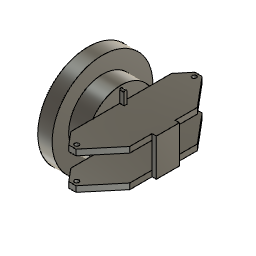
INDUSTRIAL ROBOT v3 (Autodesk Fusion 360 archive; units mm, degrees)
design "ITEM 3"
Autodesk Fusion 360 part; units mm, degrees
sketch "Sketch1" plane through (0, 0, 0) normal (1, 0, 0) x (0, 1, 0)
  circle A0 centre (0, 0) radius 35
  dimension "d1" = 70
  constraint coincident A0.centre origin
  measures "d1" diameter of A0
extrude "Extrude1" add sketch "Sketch1" along normal blind 10 in component "Component"
sketch "Sketch2" plane through (10, 0, 0) normal (1, 0, 0) x (0, 1, 0)
  circle A0 centre (0, 0) radius 35
  circle A1 centre (0, 0) radius 23.5
  dimension "d4" = 47
  constraint coincident A0.centre A1.centre
  measures "d4" diameter of A1
extrude "Extrude2" add sketch "Sketch2" along normal blind 13 contours A1 in component "Component"
ref_plane "WorkPlane1" through (0, 0, 13) normal (0, 0, 1) x (1, 0, 0)
sketch "Sketch3" plane through (0, 0, 13) normal (0, 0, 1) x (1, 0, 0)
  line L0 (23, 0) -> (23, -35)
  line L1 (23, -35) -> (23, -45)
  line L2 (23, -35) -> (30.3921, -43.8095)
  line L3 (23, -35) -> (34.5, -35) construction
  line L4 (23, 0) -> (60, 0)
  line L5 (23, -23.4992) -> (67, -23.4992)
  line L6 (30.3921, -43.8095) -> (35.3921, -43.8095)
  line L7 (35.3921, -43.8095) -> (52.4344, -23.4992)
  line L8 (35.3921, -43.8095) -> (45, -43.8095)
  line L9 (52.4344, -23.4992) -> (52.4344, 0)
  line L10 (23, 0) -> (23, 35)
  line L11 (23, 35) -> (30.3921, 43.8095)
  line L12 (30.3921, 43.8095) -> (35.3921, 43.8095)
  line L13 (52.4344, 23.4992) -> (52.4344, 0)
  line L14 (35.3921, 43.8095) -> (52.4344, 23.4992)
  dimension "d8" = 35
  dimension "d9" = 10
  dimension "d10" = 50
  dimension "d11" = 11.5
  dimension "d13" = 37
  dimension "d14" = 44
  dimension "d15" = 5
  dimension "d16" = 50
  constraint vertical L0
  constraint parallel L0 L1
  constraint horizontal L3
  constraint perpendicular L0 L4
  constraint coincident L0 L5.start
  constraint perpendicular L0 L5
  constraint horizontal L6
  constraint coincident L5 L7.end
  constraint parallel L5 L8
  constraint coincident L4 L9.end
  constraint perpendicular L4 L9
  constraint symmetric L0.start L4 L10.start
  constraint symmetric L0.end L4 L10.end
  constraint symmetric L2.end L4 L11.end
  constraint symmetric L4 L6.end L12.end
  constraint symmetric L4 L7.end L13.start
  constraint symmetric L4 L9.end L13.end
  measures "d8" distance of L0.start L0.end
  measures "d9" distance of L0.end L1.end
  measures "d10" angle of L2 L3
  measures "d11" distance of L0.end L2.end
  measures "d13" distance of L0.start L4.end
  measures "d14" distance of L5.start L5.end
  measures "d15" distance of L2.end L6.end
  measures "d16" angle of L7 L8
extrude "Extrude3" add sketch "Sketch3" against normal blind 4 in component "Component"
sketch "Sketch4" plane through (0, 0, 13) normal (0, 0, 1) x (-1, 0, 0)
  line L0 (-23, -35) -> (-23, -19.5768)
  line L1 (-23, -19.5768) -> (-23, 19.5768)
  line L2 (-23, 19.5768) -> (-23, 35)
  line L3 (-23, 35) -> (-30.3921, 43.8095)
  line L4 (-30.3921, 43.8095) -> (-35.3921, 43.8095)
  line L5 (-35.3921, 43.8095) -> (-52.4344, 23.4992)
  line L6 (-52.4344, 23.4992) -> (-52.4344, -23.4992)
  line L7 (-52.4344, -23.4992) -> (-35.3921, -43.8095)
  line L8 (-35.3921, -43.8095) -> (-30.3921, -43.8095)
  line L9 (-30.3921, -43.8095) -> (-23, -35)
  line L10 (-32.8921, 43.8095) -> (-32.8921, 40.8095)
  circle A0 centre (-32.8921, 40.8095) radius 1.5
  dimension "d19" = 3
  dimension "d20" = 3
  constraint midpoint L4 L10.start
  constraint perpendicular L4 L10
  constraint coincident L10.end A0.centre
  measures "d19" distance of L10.start L10.end
  measures "d20" diameter of A0
extrude "Extrude4" cut sketch "Sketch4" against normal blind 7 contours A0 in component "Component"
mirror "Mirror1" about plane through (0, 0, 0) normal (0, 1, 0) of "Extrude4" in component "Component"
mirror "Mirror2" about plane through (0, 0, 0) normal (0, 0, 1) of "Extrude3", "Extrude4", "Mirror1" in component "Component"
sketch "Sketch5" plane through (23, 0, 0) normal (1, 0, 0) x (0, 1, 0)
  line L0 (-19.5768, 13) -> (19.5768, 13)
  arc A0 (19.5768, 13) -> (-19.5768, 13) centre (0, 0) ccw
  line L1 (0, 13) -> (0, 23.5)
  line L2 (0, 13) -> (-1, 13)
  line L3 (-1, 13) -> (-1, 22)
  line L4 (-1, 22) -> (1, 22)
  line L5 (1, 22) -> (1, 13)
  constraint midpoint L0 L1.start
  constraint midpoint A0 L1.end
  constraint coincident L0 L2.end
  constraint perpendicular L2 L3
  constraint perpendicular L1 L4
  constraint coincident L0 L5.end
  constraint perpendicular L0 L5
extrude "Extrude5" add sketch "Sketch5" along normal blind 3 contours L0 L1 L2 L3 L4 | L0 L1 L4 L5 in component "Component"
fillet "Fillet1" radius 1 2 edges at (24.5, 1, 22) (24.5, -1, 22) in component "Component"
mirror "Mirror3" about plane through (0, 0, 0) normal (0, 0, 1) of "Extrude5", "Fillet1" in component "Component"
sketch "Sketch6" plane through (52.4344, 0, 0) normal (1, 0, 0) x (0, 1, 0)
  line L0 (23.4992, 13) -> (-23.4992, 13)
  line L1 (-23.4992, 13) -> (-23.4992, 9)
  line L2 (-23.4992, 9) -> (23.4992, 9)
  line L3 (23.4992, 9) -> (23.4992, 13)
  line L4 (8, -13) -> (-8, -13)
  line L5 (-8, -13) -> (-8, 13)
  line L6 (-8, 13) -> (8, 13)
  line L7 (8, 13) -> (8, -13)
  line L8 (8, -13) -> (-8, 13) construction
  line L9 (-8, -13) -> (8, 13) construction
  constraint horizontal L4
  constraint perpendicular L4 L5
  constraint parallel L4 L6
  constraint parallel L5 L7
  constraint coincident L8 origin
  constraint coincident L9 origin
extrude "Extrude6" add sketch "Sketch6" along normal blind 3 contours L0 L2 L5 L6 L7 | L2 L4 L5 L7 in component "Component"
sketch "Sketch7" plane through (0, 0, 0) normal (-1, 0, 0) x (0, -1, 0)
  circle A0 centre (0, 0) radius 35
  circle A1 centre (0, 0) radius 10
  dimension "d35" = 20
  constraint coincident A0.centre A1.centre
  measures "d35" diameter of A1
extrude "Extrude7" cut sketch "Sketch7" against normal blind 10 contours A1 in component "Component"
component "Component" placed x (1, 0, 0) y (0, 1, 0) z (0, 0, 1) at (0, 0, 0)

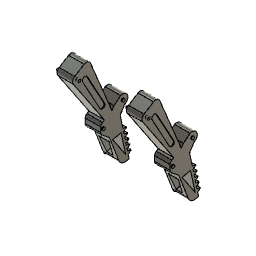
design "JAW FINAL"
Autodesk Fusion 360 part; units mm, degrees
sketch "Sketch1" plane through (0, 0, 0) normal (1, 0, 0) x (0, 1, 0)
  line L0 (308.6071, 26.1218) -> (329.0653, 38.6702)
  line L1 (329.0653, 38.6702) -> (356.1703, -26.9523)
  line L2 (364.0358, -80.7741) -> (365.4972, -87.6198)
  line L3 (365.4972, -87.6198) -> (376.2548, -85.3234)
  line L4 (376.2548, -85.3234) -> (365.8164, -36.4251)
  line L5 (365.8164, -36.4251) -> (371.2115, -28.0053)
  line L6 (308.6071, 26.1218) -> (347.5605, -32.0386)
  line L7 (356.1703, -26.9523) -> (347.5605, -32.0386)
  line L8 (347.5605, -32.0386) -> (343.2556, -34.5818)
  line L9 (343.2556, -34.5818) -> (343.2556, -44.5818)
  line L10 (343.2556, -44.5818) -> (353.387, -52.7276)
  line L11 (343.2556, -44.5818) -> (352.5031, -44.5818) construction
  line L12 (353.387, -52.7276) -> (364.0358, -80.7741)
  line L13 (356.1703, -26.9523) -> (358.6771, -23.3241)
  line L14 (358.6771, -23.3241) -> (366.4246, -17.0014)
  arc A0 (371.2115, -28.0053) -> (363.9076, -19.0555) centre (368.8181, -22.5033) ccw
  dimension "d6" = 70
  dimension "d7" = 24
  dimension "d8" = 71
  dimension "d10" = 10
  dimension "d11" = 5
  dimension "d12" = 10
  dimension "d13" = 13
  dimension "d14" = 38.8
  dimension "d15" = 30
  dimension "d16" = 7
  dimension "d17" = 11
  dimension "d18" = 50
  dimension "d19" = 10
  dimension "d20" = 4.41
  dimension "d21" = 10
  dimension "d22" = 12
  constraint perpendicular L2 L3
  constraint perpendicular L3 L4
  constraint parallel L7 L8
  constraint vertical L9
  constraint horizontal L11
  constraint coincident L14.end A0
  constraint coincident L14 A0.end
  measures "d6" distance of L0.start L6.end
  measures "d7" distance of L0.start L0.end
  measures "d8" distance of L0.end L1.end
  measures "d10" distance of L1.end L6.end
  measures "d11" distance of L6.end L8.end
  measures "d12" distance of L8.end L9.end
  measures "d13" distance of L9.end L10.end
  measures "d14" angle of L10 L11
  measures "d15" distance of L2.start L10.end
  measures "d16" distance of L2.start L2.end
  measures "d17" distance of L2.end L3.end
  measures "d18" distance of L3.end L4.end
  measures "d19" distance of L4.end L5.end
  measures "d20" distance of L1.end L13.end
  measures "d21" distance of L13.end L14.end
  measures "d22" distance of L5.end L14.end
extrude "Extrude1" add sketch "Sketch1" along normal mid plane 18 contours L0 L1 L6 L7 | L2 L3 L4 L5 L7 L8 L9 L10 L12 L13 L14 A0 in component "Component"
sketch "Sketch2" plane through (-9, 0, 0) normal (-1, 0, 0) x (0, -1, 0)
  line L0 (-347.5605, -32.0386) -> (-308.6071, 26.1218)
  line L1 (-308.6071, 26.1218) -> (-329.0653, 38.6702)
  line L2 (-329.0653, 38.6702) -> (-356.1703, -26.9523)
  line L3 (-356.1703, -26.9523) -> (-358.6771, -23.3241)
  line L4 (-358.6771, -23.3241) -> (-366.4246, -17.0014)
  arc A0 (-366.4246, -17.0014) -> (-371.2115, -28.0053) centre (-368.8181, -22.5033) ccw
  line L5 (-371.2115, -28.0053) -> (-365.8164, -36.4251)
  line L6 (-365.8164, -36.4251) -> (-376.2548, -85.3234)
  line L7 (-376.2548, -85.3234) -> (-365.4972, -87.6198)
  line L8 (-365.4972, -87.6198) -> (-364.0358, -80.7741)
  line L9 (-364.0358, -80.7741) -> (-353.387, -52.7276)
  line L10 (-353.387, -52.7276) -> (-343.2556, -44.5818)
  line L11 (-343.2556, -44.5818) -> (-343.2556, -34.5818)
  line L12 (-343.2556, -34.5818) -> (-347.5605, -32.0386)
sketch "Sketch3" plane through (9, 0, 0) normal (1, 0, 0) x (0, 1, 0)
  line L0 (308.6071, 26.1218) -> (347.5605, -32.0386)
  line L1 (347.5605, -32.0386) -> (343.2556, -34.5818)
  line L2 (343.2556, -34.5818) -> (343.2556, -44.5818)
  line L3 (343.2556, -44.5818) -> (353.387, -52.7276)
  line L4 (353.387, -52.7276) -> (364.0358, -80.7741)
  line L5 (364.0358, -80.7741) -> (365.4972, -87.6198)
  line L6 (365.4972, -87.6198) -> (376.2548, -85.3234)
  line L7 (376.2548, -85.3234) -> (365.8164, -36.4251)
  line L8 (365.8164, -36.4251) -> (371.2115, -28.0053)
  arc A0 (371.2115, -28.0053) -> (366.4246, -17.0014) centre (368.8181, -22.5033) ccw
  line L9 (366.4246, -17.0014) -> (358.6771, -23.3241)
  line L10 (358.6771, -23.3241) -> (356.1703, -26.9523)
  line L11 (356.1703, -26.9523) -> (329.0653, 38.6702)
  line L12 (329.0653, 38.6702) -> (308.6071, 26.1218)
  line L13 (364.0358, -80.7741) -> (372.1529, -79.0413)
  line L14 (372.1529, -79.0413) -> (366.9337, -54.5922)
  line L15 (372.1529, -79.0413) -> (366.9337, -54.5922)
  line L16 (366.9337, -54.5922) -> (357.1541, -56.6798)
  line L17 (357.1541, -56.6798) -> (372.1529, -79.0413)
  dimension "d25" = 90
  dimension "d26" = 25
  dimension "d28" = 2.7
  dimension "d29" = 10
  constraint coincident L4.end L5.start
  constraint perpendicular L5 L13
  constraint perpendicular L14 L16
  measures "d25" angle of L13 L14
  measures "d26" distance of L13.end L14.end
  measures "d28" distance of L7 L15
  measures "d29" distance of L14.end L16.end
extrude "Extrude2" cut sketch "Sketch3" against normal blind 68 contours L14 L15 L16 L17 in component "Component"
sketch "Sketch4" plane through (9, 0, 0) normal (1, 0, 0) x (0, 1, 0)
  line L0 (366.9337, -54.5922) -> (372.1529, -79.0413)
  line L1 (372.1529, -79.0413) -> (357.1541, -56.6798)
  line L2 (357.1541, -56.6798) -> (366.9337, -54.5922)
  line L3 (308.6071, 26.1218) -> (347.5605, -32.0386)
  line L4 (347.5605, -32.0386) -> (343.2556, -34.5818)
  line L5 (343.2556, -34.5818) -> (343.2556, -44.5818)
  line L6 (343.2556, -44.5818) -> (353.387, -52.7276)
  line L7 (353.387, -52.7276) -> (364.0358, -80.7741)
  line L8 (364.0358, -80.7741) -> (365.4972, -87.6198)
  line L9 (365.4972, -87.6198) -> (376.2548, -85.3234)
  line L10 (376.2548, -85.3234) -> (365.8164, -36.4251)
  line L11 (365.8164, -36.4251) -> (371.2115, -28.0053)
  arc A0 (371.2115, -28.0053) -> (366.4246, -17.0014) centre (368.8181, -22.5033) ccw
  line L12 (366.4246, -17.0014) -> (358.6771, -23.3241)
  line L13 (358.6771, -23.3241) -> (356.1703, -26.9523)
  line L14 (356.1703, -26.9523) -> (329.0653, 38.6702)
  line L15 (329.0653, 38.6702) -> (308.6071, 26.1218)
  line L16 (376.2548, -85.3234) -> (375.2109, -80.4336)
  line L17 (375.2109, -80.4336) -> (374.3759, -76.5217)
  line L18 (374.7934, -78.4776) -> (378.7053, -77.6426)
  line L19 (378.7053, -77.6426) -> (374.3759, -76.5217)
  line L20 (375.2109, -80.4336) -> (378.7053, -77.6426)
  line L21 (373.854, -74.0768) -> (377.3483, -71.2858)
  line L22 (373.4364, -72.1208) -> (377.3483, -71.2858)
  line L23 (377.3483, -71.2858) -> (373.0189, -70.1649)
  line L24 (373.854, -74.0768) -> (373.0189, -70.1649)
  line L25 (372.497, -67.72) -> (375.9913, -64.929)
  line L26 (372.0794, -65.7641) -> (375.9913, -64.929)
  line L27 (375.9913, -64.929) -> (371.6619, -63.8081)
  line L28 (372.497, -67.72) -> (371.6619, -63.8081)
  line L29 (371.14, -61.3632) -> (374.6343, -58.5722)
  line L30 (370.7225, -59.4073) -> (374.6343, -58.5722)
  line L31 (374.6343, -58.5722) -> (370.3049, -57.4514)
  line L32 (371.14, -61.3632) -> (370.3049, -57.4514)
  line L33 (369.783, -55.0065) -> (373.2773, -52.2155)
  line L34 (369.3655, -53.0505) -> (373.2773, -52.2155)
  line L35 (373.2773, -52.2155) -> (368.9479, -51.0946)
  line L36 (369.783, -55.0065) -> (368.9479, -51.0946)
  dimension "d32" = 5
  dimension "d33" = 4
  dimension "d34" = 4
  dimension "d37" = 26
  dimension "d38" = 0
  constraint coincident L9.end L10.start
  constraint perpendicular L9 L16
  constraint perpendicular L9 L17
  constraint midpoint L17 L18.start
  constraint perpendicular L17 L18
  measures "d32" distance of L9.end L16.end
  measures "d33" distance of L16.end L17.end
  measures "d34" distance of L18.start L18.end
extrude "Extrude3" add sketch "Sketch4" against normal up to surface (18 mm away) contours L10 L34 L35 L36 | L10 L17 L18 L20 | L10 L33 L34 L36 | L10 L17 L18 L19 | L10 L30 L31 L32 | L10 L21 L22 L24 | L10 L29 L30 L32 | L10 L22 L23 L24 | L10 L26 L27 L28 | L10 L25 L26 L28 in component "Component"
fillet "Fillet1" radius 5 2 edges at (0, 308.6071, 26.1218) (0, 329.0653, 38.6702) in component "Component"
fillet "Fillet2" radius 7.5 1 edges at (0, 365.4972, -87.6198) in component "Component"
fillet "Fillet3" radius 4 2 edges at (0, 343.2556, -44.5818) (0, 343.2556, -34.5818) in component "Component"
sketch "Sketch5" plane through (9, 0, 0) normal (1, 0, 0) x (0, 1, 0)
  arc A0 (345.221, -33.4207) -> (343.2556, -36.8646) centre (347.2556, -36.8646) ccw
  line L0 (343.2556, -36.8646) -> (343.2556, -42.6653)
  arc A1 (343.2556, -42.6653) -> (344.7491, -45.7827) centre (347.2556, -42.6653) ccw
  line L1 (344.7491, -45.7827) -> (353.387, -52.7276)
  line L2 (353.387, -52.7276) -> (364.0358, -80.7741)
  arc A2 (364.0358, -80.7741) -> (372.8156, -86.0576) centre (371.2498, -78.7228) ccw
  line L3 (372.8156, -86.0576) -> (376.2548, -85.3234)
  line L4 (376.2548, -85.3234) -> (375.2109, -80.4336)
  line L5 (375.2109, -80.4336) -> (378.7053, -77.6426)
  line L6 (378.7053, -77.6426) -> (374.3759, -76.5217)
  line L7 (374.3759, -76.5217) -> (373.854, -74.0768)
  line L8 (373.854, -74.0768) -> (377.3483, -71.2858)
  line L9 (377.3483, -71.2858) -> (373.0189, -70.1649)
  line L10 (373.0189, -70.1649) -> (372.497, -67.72)
  line L11 (372.497, -67.72) -> (375.9913, -64.929)
  line L12 (375.9913, -64.929) -> (371.6619, -63.8081)
  line L13 (371.6619, -63.8081) -> (371.14, -61.3632)
  line L14 (371.14, -61.3632) -> (374.6343, -58.5722)
  line L15 (374.6343, -58.5722) -> (370.3049, -57.4514)
  line L16 (370.3049, -57.4514) -> (369.783, -55.0065)
  line L17 (369.783, -55.0065) -> (373.2773, -52.2155)
  line L18 (373.2773, -52.2155) -> (368.9479, -51.0946)
  line L19 (368.9479, -51.0946) -> (365.8164, -36.4251)
  line L20 (365.8164, -36.4251) -> (371.2115, -28.0053)
  arc A3 (371.2115, -28.0053) -> (366.4246, -17.0014) centre (368.8181, -22.5033) ccw
  line L21 (366.4246, -17.0014) -> (358.6771, -23.3241)
  line L22 (358.6771, -23.3241) -> (356.1703, -26.9523)
  line L23 (356.1703, -26.9523) -> (331.3034, 33.2516)
  arc A4 (331.3034, 33.2516) -> (324.0678, 35.6049) centre (326.6821, 31.3428) ccw
  line L24 (324.0678, 35.6049) -> (313.043, 28.8426)
  arc A5 (313.043, 28.8426) -> (311.5029, 21.7981) centre (315.6572, 24.5805) ccw
  line L25 (311.5029, 21.7981) -> (347.5605, -32.0386)
  line L26 (347.5605, -32.0386) -> (345.221, -33.4207)
  line L27 (366.9337, -54.5922) -> (372.1529, -79.0413)
  line L28 (372.1529, -79.0413) -> (357.1541, -56.6798)
  line L29 (357.1541, -56.6798) -> (366.9337, -54.5922)
  circle A6 centre (314.3303, 24.5805) radius 1.5
  dimension "d49" = 3
  measures "d49" diameter of A6
extrude "Extrude4" cut sketch "Sketch5" against normal blind 29 contours A6 in component "Component"
sketch "Sketch6" plane through (0, 291.3636, 110.6267) normal (0, -0.934881, -0.354961) x (1, 0, 0)
  line L0 (-9, -204.7328) -> (9, -204.7328)
  line L1 (9, -204.7328) -> (9, -174.7328)
  line L2 (9, -174.7328) -> (-9, -174.7328)
  line L3 (-9, -174.7328) -> (-9, -204.7328)
  line L4 (-6, -182.1738) -> (6, -182.1738)
  line L5 (-7, -201.7782) -> (3.528, -201.7782)
  line L6 (3.528, -201.7782) -> (6, -182.1738)
  line L7 (-6, -182.1738) -> (-3.4614, -201.7782)
  dimension "d52" = 3
  dimension "d53" = 3
  dimension "d54" = 7.441
  constraint horizontal L4
  constraint horizontal L5
  constraint coincident L5 L7.end
  measures "d52" distance of L1 L4.end
  measures "d53" distance of L3 L4.start
  measures "d54" distance of L2 L4
extrude "Extrude5" cut sketch "Sketch6" against normal blind 8 contours L4 L5 L6 L7 in component "Component"
sketch "Sketch7" plane through (9, 0, 0) normal (1, 0, 0) x (0, 1, 0)
  circle A0 centre (314.3303, 24.5805) radius 1.5
  arc A1 (345.221, -33.4207) -> (343.2556, -36.8646) centre (347.2556, -36.8646) ccw
  line L0 (343.2556, -36.8646) -> (343.2556, -42.6653)
  arc A2 (343.2556, -42.6653) -> (344.7491, -45.7827) centre (347.2556, -42.6653) ccw
  line L1 (344.7491, -45.7827) -> (353.387, -52.7276)
  line L2 (353.387, -52.7276) -> (364.0358, -80.7741)
  arc A3 (364.0358, -80.7741) -> (372.8156, -86.0576) centre (371.2498, -78.7228) ccw
  line L3 (372.8156, -86.0576) -> (376.2548, -85.3234)
  line L4 (376.2548, -85.3234) -> (375.2109, -80.4336)
  line L5 (375.2109, -80.4336) -> (378.7053, -77.6426)
  line L6 (378.7053, -77.6426) -> (374.3759, -76.5217)
  line L7 (374.3759, -76.5217) -> (373.854, -74.0768)
  line L8 (373.854, -74.0768) -> (377.3483, -71.2858)
  line L9 (377.3483, -71.2858) -> (373.0189, -70.1649)
  line L10 (373.0189, -70.1649) -> (372.497, -67.72)
  line L11 (372.497, -67.72) -> (375.9913, -64.929)
  line L12 (375.9913, -64.929) -> (371.6619, -63.8081)
  line L13 (371.6619, -63.8081) -> (371.14, -61.3632)
  line L14 (371.14, -61.3632) -> (374.6343, -58.5722)
  line L15 (374.6343, -58.5722) -> (370.3049, -57.4514)
  line L16 (370.3049, -57.4514) -> (369.783, -55.0065)
  line L17 (369.783, -55.0065) -> (373.2773, -52.2155)
  line L18 (373.2773, -52.2155) -> (368.9479, -51.0946)
  line L19 (368.9479, -51.0946) -> (365.8164, -36.4251)
  line L20 (365.8164, -36.4251) -> (371.2115, -28.0053)
  arc A4 (371.2115, -28.0053) -> (366.4246, -17.0014) centre (368.8181, -22.5033) ccw
  line L21 (366.4246, -17.0014) -> (358.6771, -23.3241)
  line L22 (358.6771, -23.3241) -> (356.1703, -26.9523)
  line L23 (356.1703, -26.9523) -> (331.3034, 33.2516)
  arc A5 (331.3034, 33.2516) -> (324.0678, 35.6049) centre (326.6821, 31.3428) ccw
  line L24 (324.0678, 35.6049) -> (313.043, 28.8426)
  arc A6 (313.043, 28.8426) -> (311.5029, 21.7981) centre (315.6572, 24.5805) ccw
  line L25 (311.5029, 21.7981) -> (347.5605, -32.0386)
  line L26 (347.5605, -32.0386) -> (345.221, -33.4207)
  line L27 (366.9337, -54.5922) -> (372.1529, -79.0413)
  line L28 (372.1529, -79.0413) -> (357.1541, -56.6798)
  line L29 (357.1541, -56.6798) -> (366.9337, -54.5922)
  circle A7 centre (368.8181, -22.5033) radius 1.75
  circle A8 centre (345.9618, -39.765) radius 1.75
  dimension "d57" = 3.5
  dimension "d58" = 3.5
  constraint concentric A4 A7
  measures "d57" diameter of A7
  measures "d58" diameter of A8
extrude "Extrude6" add sketch "Sketch7" along normal blind 1 contours A7 | A8 in component "Component"
sketch "Sketch8" plane through (9, 0, 0) normal (1, 0, 0) x (0, 1, 0)
  circle A0 centre (368.8181, -22.5033) radius 1.75
  circle A1 centre (345.9618, -39.765) radius 1.75
  circle A2 centre (314.3303, 24.5805) radius 1.5
  arc A3 (345.221, -33.4207) -> (343.2556, -36.8646) centre (347.2556, -36.8646) ccw
  line L0 (343.2556, -36.8646) -> (343.2556, -42.6653)
  arc A4 (343.2556, -42.6653) -> (344.7491, -45.7827) centre (347.2556, -42.6653) ccw
  line L1 (344.7491, -45.7827) -> (353.387, -52.7276)
  line L2 (353.387, -52.7276) -> (364.0358, -80.7741)
  arc A5 (364.0358, -80.7741) -> (372.8156, -86.0576) centre (371.2498, -78.7228) ccw
  line L3 (372.8156, -86.0576) -> (376.2548, -85.3234)
  line L4 (376.2548, -85.3234) -> (375.2109, -80.4336)
  line L5 (375.2109, -80.4336) -> (378.7053, -77.6426)
  line L6 (378.7053, -77.6426) -> (374.3759, -76.5217)
  line L7 (374.3759, -76.5217) -> (373.854, -74.0768)
  line L8 (373.854, -74.0768) -> (377.3483, -71.2858)
  line L9 (377.3483, -71.2858) -> (373.0189, -70.1649)
  line L10 (373.0189, -70.1649) -> (372.497, -67.72)
  line L11 (372.497, -67.72) -> (375.9913, -64.929)
  line L12 (375.9913, -64.929) -> (371.6619, -63.8081)
  line L13 (371.6619, -63.8081) -> (371.14, -61.3632)
  line L14 (371.14, -61.3632) -> (374.6343, -58.5722)
  line L15 (374.6343, -58.5722) -> (370.3049, -57.4514)
  line L16 (370.3049, -57.4514) -> (369.783, -55.0065)
  line L17 (369.783, -55.0065) -> (373.2773, -52.2155)
  line L18 (373.2773, -52.2155) -> (368.9479, -51.0946)
  line L19 (368.9479, -51.0946) -> (365.8164, -36.4251)
  line L20 (365.8164, -36.4251) -> (371.2115, -28.0053)
  arc A6 (371.2115, -28.0053) -> (366.4246, -17.0014) centre (368.8181, -22.5033) ccw
  line L21 (366.4246, -17.0014) -> (358.6771, -23.3241)
  line L22 (358.6771, -23.3241) -> (356.1703, -26.9523)
  line L23 (356.1703, -26.9523) -> (331.3034, 33.2516)
  arc A7 (331.3034, 33.2516) -> (324.0678, 35.6049) centre (326.6821, 31.3428) ccw
  line L24 (324.0678, 35.6049) -> (313.043, 28.8426)
  arc A8 (313.043, 28.8426) -> (311.5029, 21.7981) centre (315.6572, 24.5805) ccw
  line L25 (311.5029, 21.7981) -> (347.5605, -32.0386)
  line L26 (347.5605, -32.0386) -> (345.221, -33.4207)
  line L27 (366.9337, -54.5922) -> (372.1529, -79.0413)
  line L28 (372.1529, -79.0413) -> (357.1541, -56.6798)
  line L29 (357.1541, -56.6798) -> (366.9337, -54.5922)
  line L30 (322.3738, 18.5661) -> (342.5242, -18.3398)
  arc A9 (342.5242, -18.3398) -> (347.7767, -15.4719) centre (345.1504, -16.9058) ccw
  line L31 (347.7767, -15.4719) -> (327.6262, 21.4339)
  arc A10 (327.6262, 21.4339) -> (322.3738, 18.5661) centre (325, 20) ccw
  line L32 (325, 20) -> (345.1504, -16.9058) construction
  constraint tangent L30 A9
  constraint tangent A9 L31
  constraint parallel L30 L31
  constraint tangent L31 A10
  constraint tangent L30 A10
extrude "Extrude7" cut sketch "Sketch8" against normal blind 1 contours L30 A9 L31 A10 in component "Component"
mirror "Mirror1" about plane through (0, 344.5115, -25.3555) normal (1, 0, 0) of "Extrude6", "Extrude7" in component "Component"
sketch "Sketch9" plane through (9, 0, 0) normal (1, 0, 0) x (0, 1, 0)
  line L0 (342.5242, -18.3398) -> (322.3738, 18.5661)
  arc A0 (327.6262, 21.4339) -> (322.3738, 18.5661) centre (325, 20) ccw
  line L1 (327.6262, 21.4339) -> (347.7767, -15.4719)
  arc A1 (342.5242, -18.3398) -> (347.7767, -15.4719) centre (345.1504, -16.9058) ccw
  circle A2 centre (368.8181, -22.5033) radius 1.75
  circle A3 centre (345.9618, -39.765) radius 1.75
  circle A4 centre (314.3303, 24.5805) radius 1.5
  arc A5 (345.221, -33.4207) -> (343.2556, -36.8646) centre (347.2556, -36.8646) ccw
  line L2 (343.2556, -36.8646) -> (343.2556, -42.6653)
  arc A6 (343.2556, -42.6653) -> (344.7491, -45.7827) centre (347.2556, -42.6653) ccw
  line L3 (344.7491, -45.7827) -> (353.387, -52.7276)
  line L4 (353.387, -52.7276) -> (364.0358, -80.7741)
  arc A7 (364.0358, -80.7741) -> (372.8156, -86.0576) centre (371.2498, -78.7228) ccw
  line L5 (372.8156, -86.0576) -> (376.2548, -85.3234)
  line L6 (376.2548, -85.3234) -> (375.2109, -80.4336)
  line L7 (375.2109, -80.4336) -> (378.7053, -77.6426)
  line L8 (378.7053, -77.6426) -> (374.3759, -76.5217)
  line L9 (374.3759, -76.5217) -> (373.854, -74.0768)
  line L10 (373.854, -74.0768) -> (377.3483, -71.2858)
  line L11 (377.3483, -71.2858) -> (373.0189, -70.1649)
  line L12 (373.0189, -70.1649) -> (372.497, -67.72)
  line L13 (372.497, -67.72) -> (375.9913, -64.929)
  line L14 (375.9913, -64.929) -> (371.6619, -63.8081)
  line L15 (371.6619, -63.8081) -> (371.14, -61.3632)
  line L16 (371.14, -61.3632) -> (374.6343, -58.5722)
  line L17 (374.6343, -58.5722) -> (370.3049, -57.4514)
  line L18 (370.3049, -57.4514) -> (369.783, -55.0065)
  line L19 (369.783, -55.0065) -> (373.2773, -52.2155)
  line L20 (373.2773, -52.2155) -> (368.9479, -51.0946)
  line L21 (368.9479, -51.0946) -> (365.8164, -36.4251)
  line L22 (365.8164, -36.4251) -> (371.2115, -28.0053)
  arc A8 (371.2115, -28.0053) -> (366.4246, -17.0014) centre (368.8181, -22.5033) ccw
  line L23 (366.4246, -17.0014) -> (358.6771, -23.3241)
  line L24 (358.6771, -23.3241) -> (356.1703, -26.9523)
  line L25 (356.1703, -26.9523) -> (331.3034, 33.2516)
  arc A9 (331.3034, 33.2516) -> (324.0678, 35.6049) centre (326.6821, 31.3428) ccw
  line L26 (324.0678, 35.6049) -> (313.043, 28.8426)
  arc A10 (313.043, 28.8426) -> (311.5029, 21.7981) centre (315.6572, 24.5805) ccw
  line L27 (311.5029, 21.7981) -> (347.5605, -32.0386)
  line L28 (347.5605, -32.0386) -> (345.221, -33.4207)
  line L29 (366.9337, -54.5922) -> (372.1529, -79.0413)
  line L30 (372.1529, -79.0413) -> (357.1541, -56.6798)
  line L31 (357.1541, -56.6798) -> (366.9337, -54.5922)
  circle A11 centre (314.3303, 24.5805) radius 1.5
  constraint concentric A4 A11
extrude "Extrude8" add sketch "Sketch9" against normal blind 21 contours A4 A11 in component "Component"
sketch "Sketch10" plane through (9, 0, 0) normal (1, 0, 0) x (0, 1, 0)
  line L0 (342.5242, -18.3398) -> (322.3738, 18.5661)
  arc A0 (327.6262, 21.4339) -> (322.3738, 18.5661) centre (325, 20) ccw
  line L1 (327.6262, 21.4339) -> (347.7767, -15.4719)
  arc A1 (342.5242, -18.3398) -> (347.7767, -15.4719) centre (345.1504, -16.9058) ccw
  circle A2 centre (368.8181, -22.5033) radius 1.75
  circle A3 centre (345.9618, -39.765) radius 1.75
  arc A4 (345.221, -33.4207) -> (343.2556, -36.8646) centre (347.2556, -36.8646) ccw
  line L2 (343.2556, -36.8646) -> (343.2556, -42.6653)
  arc A5 (343.2556, -42.6653) -> (344.7491, -45.7827) centre (347.2556, -42.6653) ccw
  line L3 (344.7491, -45.7827) -> (353.387, -52.7276)
  line L4 (353.387, -52.7276) -> (364.0358, -80.7741)
  arc A6 (364.0358, -80.7741) -> (372.8156, -86.0576) centre (371.2498, -78.7228) ccw
  line L5 (372.8156, -86.0576) -> (376.2548, -85.3234)
  line L6 (376.2548, -85.3234) -> (375.2109, -80.4336)
  line L7 (375.2109, -80.4336) -> (378.7053, -77.6426)
  line L8 (378.7053, -77.6426) -> (374.3759, -76.5217)
  line L9 (374.3759, -76.5217) -> (373.854, -74.0768)
  line L10 (373.854, -74.0768) -> (377.3483, -71.2858)
  line L11 (377.3483, -71.2858) -> (373.0189, -70.1649)
  line L12 (373.0189, -70.1649) -> (372.497, -67.72)
  line L13 (372.497, -67.72) -> (375.9913, -64.929)
  line L14 (375.9913, -64.929) -> (371.6619, -63.8081)
  line L15 (371.6619, -63.8081) -> (371.14, -61.3632)
  line L16 (371.14, -61.3632) -> (374.6343, -58.5722)
  line L17 (374.6343, -58.5722) -> (370.3049, -57.4514)
  line L18 (370.3049, -57.4514) -> (369.783, -55.0065)
  line L19 (369.783, -55.0065) -> (373.2773, -52.2155)
  line L20 (373.2773, -52.2155) -> (368.9479, -51.0946)
  line L21 (368.9479, -51.0946) -> (365.8164, -36.4251)
  line L22 (365.8164, -36.4251) -> (371.2115, -28.0053)
  arc A7 (371.2115, -28.0053) -> (366.4246, -17.0014) centre (368.8181, -22.5033) ccw
  line L23 (366.4246, -17.0014) -> (358.6771, -23.3241)
  line L24 (358.6771, -23.3241) -> (356.1703, -26.9523)
  line L25 (356.1703, -26.9523) -> (331.3034, 33.2516)
  arc A8 (331.3034, 33.2516) -> (324.0678, 35.6049) centre (326.6821, 31.3428) ccw
  line L26 (324.0678, 35.6049) -> (313.043, 28.8426)
  arc A9 (313.043, 28.8426) -> (311.5029, 21.7981) centre (315.6572, 24.5805) ccw
  line L27 (311.5029, 21.7981) -> (347.5605, -32.0386)
  line L28 (347.5605, -32.0386) -> (345.221, -33.4207)
  line L29 (366.9337, -54.5922) -> (372.1529, -79.0413)
  line L30 (372.1529, -79.0413) -> (357.1541, -56.6798)
  line L31 (357.1541, -56.6798) -> (366.9337, -54.5922)
  circle A10 centre (315.6572, 24.5805) radius 1.5
  dimension "d67" = 3
  constraint concentric A9 A10
  measures "d67" diameter of A10
extrude "Extrude9" add sketch "Sketch10" along normal blind 3 contours A10 in component "Component"
sketch "Sketch11" plane through (-12, 0, 0) normal (-1, 0, 0) x (0, -1, 0)
  circle A0 centre (-314.3303, 24.5805) radius 1.5
component "Component" placed x (1, 0, 0) y (0, 1, 0) z (0, 0, 1) at (0, 0, 0)
component "Component" placed x (1, 0, 0) y (0, 1, 0) z (0, 0, 1) at (52.854, 27.602, -25.252)

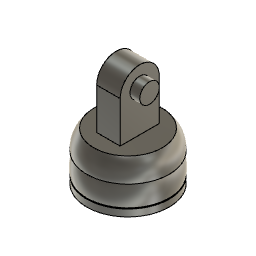
design "ITEM 2"
Autodesk Fusion 360 part; units mm, degrees
sketch "Sketch1" plane through (0, 0, 0) normal (0, 1, 0) x (1, 0, 0)
  line L0 (0, 0) -> (-35, 0)
  line L1 (0, 0) -> (0, 20)
  line L2 (0, 20) -> (-42, 20)
  arc A0 (-42, 20) -> (-35, 0) centre (-17.1273, 17.4804) ccw
  dimension "d1" = 35
  dimension "d2" = 20
  dimension "d3" = 42
  dimension "d4" = 25
  constraint coincident L0.start L1.start
  constraint horizontal L0
  constraint vertical L1
  constraint perpendicular L1 L2
  measures "d1" distance of L0.start L0.end
  measures "d2" distance of L0.start L1.end
  measures "d3" distance of L1.end L2.end
  measures "d4" radius of A0
revolve "Revolve1" add sketch "Sketch1" angle 360 about axis through (0, 0, 0) along (0, 0, -1) in component "Component"
sketch "Sketch2" plane through (0, 0, -20) normal (0, 0, -1) x (1, 0, 0)
  circle A0 centre (0, 0) radius 42
  circle A1 centre (0, 0) radius 39.5
  dimension "d6" = 79
  constraint coincident A0.centre A1.centre
  measures "d6" diameter of A1
extrude "Extrude1" add sketch "Sketch2" along normal blind 1 contours A1 in component "Component"
sketch "Sketch3" plane through (0, 0, 0) normal (1, 0, 0) x (0, 1, 0)
  line L0 (0, -21) -> (0, -41)
  line L1 (0, -41) -> (-42, -41)
  line L2 (0, -21) -> (-40, -21)
  arc A0 (-40, -21) -> (-42, -41) centre (-5.5677, -34.5432) ccw
  dimension "d9" = 20
  dimension "d10" = 42
  dimension "d11" = 40
  dimension "d12" = 37
  constraint vertical L0
  constraint perpendicular L0 L1
  constraint perpendicular L0 L2
  measures "d9" distance of L0.start L0.end
  measures "d10" distance of L0.end L1.end
  measures "d11" distance of L0.start L2.end
  measures "d12" radius of A0
revolve "Revolve2" add sketch "Sketch3" angle 360 about axis through (0, 0, -21) along (0, 0, -1) in component "Component"
sketch "Sketch4" plane through (0, 0, -41) normal (0, 0, -1) x (1, 0, 0)
  circle A0 centre (0, 0) radius 42
  circle A1 centre (0, 0) radius 41
  dimension "d14" = 82
  constraint coincident A0.centre A1.centre
  measures "d14" diameter of A1
extrude "Extrude2" add sketch "Sketch4" along normal blind 1 contours A1 in component "Component"
sketch "Sketch5" plane through (0, 0, -42) normal (0, 0, -1) x (1, 0, 0)
  circle A0 centre (0, 0) radius 41
  circle A1 centre (0, 0) radius 42
  dimension "d17" = 84
  constraint coincident A0.centre A1.centre
  measures "d17" diameter of A1
extrude "Extrude3" add sketch "Sketch5" along normal blind 7 contours A0 | A1 in component "Component"
sketch "Sketch6" plane through (0, 0, -49) normal (0, 0, -1) x (1, 0, 0)
  circle A0 centre (0, 0) radius 42
  circle A1 centre (0, 0) radius 35
  dimension "d20" = 70
  constraint coincident A0.centre A1.centre
  measures "d20" diameter of A1
extrude "Extrude4" add sketch "Sketch6" along normal blind 3 contours A1 in component "Component"
sketch "Sketch7" plane through (0, 0, -49) normal (0, 0, -1) x (1, 0, 0)
  circle A0 centre (0, 0) radius 35
  circle A1 centre (0, 0) radius 42
  line L0 (35, 0.0167) -> (42, 0.0167)
  circle A2 centre (38.5, 0.0167) radius 2.25
  circle A3 centre (38.5, 0.0167) radius 1.5
  dimension "d23" = 4.5
  dimension "d24" = 3
  constraint coincident A0 L0.start
  constraint horizontal L0
  constraint midpoint L0 A2.centre
  constraint concentric A2 A3
  measures "d23" diameter of A2
  measures "d24" diameter of A3
extrude "Extrude5" add sketch "Sketch7" along normal blind 1 contours L0 A2 A3 | L0 A2 A3 in component "Component"
pattern_circular "C-Pattern1" count 16 over 360 about axis through (0, 0, -49) along (0, 0, 1) of "Extrude5" in component "Component"
sketch "Sketch8" plane through (0, 0, 0) normal (0, 0, 1) x (-1, 0, 0)
  circle A0 centre (0, 0) radius 35
  line L0 (12, 20) -> (-12, 20)
  line L1 (-12, 20) -> (-12, -20)
  line L2 (-12, -20) -> (12, -20)
  line L3 (12, -20) -> (12, 20)
  line L4 (12, 20) -> (-12, -20) construction
  line L5 (-12, 20) -> (12, -20) construction
  dimension "d29" = 24
  dimension "d30" = 40
  constraint horizontal L0
  constraint perpendicular L0 L1
  constraint parallel L0 L2
  constraint parallel L1 L3
  constraint coincident L4 A0.centre
  constraint coincident L5 A0.centre
  constraint coincident A0.centre origin
  measures "d29" distance of L1.end L2.end
  measures "d30" distance of L0.end L1.end
extrude "Extrude6" add sketch "Sketch8" along normal blind 42 contours L0 L1 L2 L3 in component "Component"
sketch "Sketch9" plane through (12, 0, 0) normal (1, 0, 0) x (0, 1, 0)
  line L0 (-20, 0) -> (20, 0)
  line L1 (20, 0) -> (20, 42)
  line L2 (20, 42) -> (-20, 42)
  line L3 (-20, 42) -> (-20, 0)
  circle A0 centre (0, 42) radius 20
  constraint midpoint L2 A0.centre
  constraint coincident L2.end A0
extrude "Extrude7" add sketch "Sketch9" against normal blind 24 contours L2 A0 picked at (4.1566, 47.2122) in component "Component"
sketch "Sketch10" plane through (12, 0, 0) normal (1, 0, 0) x (0, 1, 0)
  line L0 (-20, 0) -> (20, 0)
  line L1 (20, 0) -> (20, 42)
  arc A0 (20, 42) -> (-20, 42) centre (0, 42) ccw
  line L2 (-20, 42) -> (-20, 0)
  circle A1 centre (0, 42) radius 10
  dimension "d35" = 20
  constraint concentric A0 A1
  measures "d35" diameter of A1
extrude "Extrude8" add sketch "Sketch10" along normal blind 10 contours A1 in component "Component"
sketch "Sketch11" plane through (0, 0, -52) normal (0, 0, -1) x (1, 0, 0)
  circle A0 centre (0, 0) radius 35
  circle A1 centre (0, 0) radius 10
  dimension "d38" = 20
  constraint coincident A0.centre A1.centre
  measures "d38" diameter of A1
extrude "Extrude9" add sketch "Sketch11" along normal blind 10 contours A1 in component "Component"
component "Component" placed x (1, 0, 0) y (0, 1, 0) z (0, 0, 1) at (0, 0, 0)
